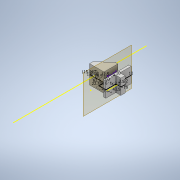
# Autodesk Inventor part: UpperObjectiveMountAssembly
Saved by Autodesk Inventor 2020 (Build 240168000, 168)
## iProperties
Created: 2017-02-08
Part Number: UpperObjectiveMountAssembly
Material: Generic
Document SubType Name: Modeling
Designer: map
Density: 1 g/cm^3
Appearance: Default
Author: map
Autodesk Inventor part; units mm, degrees
ref_plane "XZ Plane" through (0, 0, 0) normal (0, 1, 0) x (-1, 0, 0)
ref_plane "XY Plane" through (0, 0, 0) normal (0, 0, 1) x (1, 0, 0)
sketch "HolePattern" plane through (0, 0, 0) normal (0, 0, 1) x (1, 0, 0)
  arc A0 (32.9386, -36.2368) -> (4.453, -49.3983) centre (80, -175.5) ccw
  arc A1 (1.9216, -50.9498) -> (4.453, -49.3983) centre (4, -51.5) ccw
  arc A2 (1.9216, -50.9498) -> (0, -52.1752) centre (80, -175.5) ccw
  line L0 (0, -52.1752) -> (0, -56)
  line L1 (0, -56) -> (9, -56)
  line L2 (9, -56) -> (24, -56)
  line L3 (24, -56) -> (39, -56)
  line L4 (39, -56) -> (54, -56)
  line L5 (54, -56) -> (69, -56)
  line L6 (69, -56) -> (84, -56)
  line L7 (84, -56) -> (99, -56)
  line L8 (99, -56) -> (108, -56)
  line L9 (108, -56) -> (108, -52.1752)
  arc A3 (108, -52.1752) -> (106.0784, -50.9498) centre (28, -175.5) ccw
  arc A4 (103.547, -49.3983) -> (106.0784, -50.9498) centre (104, -51.5) ccw
  arc A5 (103.547, -49.3983) -> (75.0614, -36.2368) centre (28, -175.5) ccw
  arc A6 (75.0614, -26.7632) -> (75.0614, -36.2368) centre (76.6621, -31.5) ccw
  arc A7 (75.0614, -26.7632) -> (103.547, -13.6017) centre (28, 112.5) ccw
  arc A8 (106.0784, -12.0502) -> (103.547, -13.6017) centre (104, -11.5) ccw
  arc A9 (106.0784, -12.0502) -> (108, -10.8248) centre (28, 112.5) ccw
  line L10 (108, -10.8248) -> (108, 0)
  line L11 (108, 0) -> (0, 0)
  line L12 (0, 0) -> (0, -10.8248)
  arc A10 (0, -10.8248) -> (1.9216, -12.0502) centre (80, 112.5) ccw
  arc A11 (4.453, -13.6017) -> (1.9216, -12.0502) centre (4, -11.5) ccw
  arc A12 (4.453, -13.6017) -> (32.9386, -26.7632) centre (80, 112.5) ccw
  arc A13 (32.9386, -36.2368) -> (32.9386, -26.7632) centre (31.3379, -31.5) ccw
  circle A14 centre (49, -26.5) radius 1.05
  circle A15 centre (59, -36.5) radius 1.05
  circle A16 centre (54, -18.5) radius 1.05
  circle A17 centre (54, -44.5) radius 1.05
  circle A18 centre (59, -21.5) radius 0.75
  circle A19 centre (59, -26.5) radius 0.75
  circle A20 centre (59, -31.5) radius 0.75
  circle A21 centre (59, -41.5) radius 0.75
  circle A22 centre (49, -21.5) radius 0.75
  circle A23 centre (49, -31.5) radius 0.75
  circle A24 centre (49, -36.5) radius 0.75
  circle A25 centre (49, -41.5) radius 0.75
  circle A26 centre (54, -22.5) radius 1.05
  circle A27 centre (54, -40.5) radius 1.05
  circle A28 centre (74, -24) radius 1.25
  circle A29 centre (74, -39) radius 1.25
  circle A30 centre (34, -24) radius 1.25
  circle A31 centre (34, -39) radius 1.25
  circle A32 centre (72.5, -13) radius 1.3
  circle A33 centre (72.5, -50) radius 1.3
  circle A34 centre (35.5, -13) radius 1.3
  circle A35 centre (35.5, -50) radius 1.3
  circle A36 centre (54, -27) radius 1.5
  circle A37 centre (54, -36) radius 1.5
  circle A38 centre (68.5, -24) radius 1.55
  circle A39 centre (68.5, -39) radius 1.55
  circle A40 centre (39.5, -24) radius 1.55
  circle A41 centre (39.5, -39) radius 1.55
  circle A42 centre (61.5, -17) radius 2.8
  circle A43 centre (61.5, -46) radius 2.8
  circle A44 centre (46.5, -17) radius 2.8
  circle A45 centre (46.5, -46) radius 2.8
  circle A46 centre (99, -4) radius 3
  circle A47 centre (84, -4) radius 3
  circle A48 centre (69, -4) radius 3
  circle A49 centre (54, -4) radius 3
  circle A50 centre (39, -4) radius 3
  circle A51 centre (24, -4) radius 3
  circle A52 centre (9, -4) radius 3
  circle A53 centre (39, -46.5) radius 1.3
  circle A54 centre (39, -16.5) radius 1.3
  circle A55 centre (69, -46.5) radius 1.3
  circle A56 centre (69, -16.5) radius 1.3
  circle A57 centre (41.5, -44) radius 1.05
  circle A58 centre (41.5, -31.5) radius 1.05
  circle A59 centre (41.5, -19) radius 1.05
  circle A60 centre (66.5, -44) radius 1.05
  circle A61 centre (66.5, -19) radius 1.05
  circle A62 centre (66.5, -31.5) radius 1.05
  circle A63 centre (44, -41.5) radius 1.05
  circle A64 centre (44, -31.5) radius 1.05
  circle A65 centre (44, -21.5) radius 1.05
  circle A66 centre (64, -41.5) radius 1.05
  circle A67 centre (64, -21.5) radius 1.05
  circle A68 centre (64, -31.5) radius 1.05
  circle A69 centre (46, -34) radius 1
  circle A70 centre (46, -29) radius 1
  circle A71 centre (62, -34) radius 1
  circle A72 centre (62, -29) radius 1
  line L13 (59, -31.5) -> (49, -31.5) construction
  line L14 (54, -36) -> (54, -27) construction
  point P0 (54, -32.5208)
  point P1 (54, -31.5)
sketch "N-565-Profile" plane through (0, 0, 0) normal (0, 0, 1) x (1, 0, 0)
  line L0 (46.2742, 127.3015) -> (66.2742, 127.3015)
  line L1 (66.2742, 127.3015) -> (66.2742, 17.3015)
  line L2 (66.2742, 17.3015) -> (46.2742, 17.3015)
  line L3 (46.2742, 17.3015) -> (46.2742, 127.3015)
  line L4 (46.2742, 127.3015) -> (66.2742, 127.3015) construction
  line L5 (66.2742, 127.3015) -> (66.2742, 140.3015) construction
  line L6 (66.2742, 140.3015) -> (46.2742, 140.3015) construction
  line L7 (46.2742, 140.3015) -> (46.2742, 127.3015) construction
  line L8 (46.2742, 17.3015) -> (66.2742, 17.3015) construction
  line L9 (66.2742, 17.3015) -> (66.2742, 4.3015) construction
  line L10 (66.2742, 4.3015) -> (46.2742, 4.3015) construction
  line L11 (46.2742, 4.3015) -> (46.2742, 17.3015) construction
  point P0 (57.1314, 70.3586)
  point P1 (46.2742, 72.3015)
  dimension "d14" = 20
  dimension "d15" = 110
  dimension "d16" = 13
  dimension "d17" = 13
  measures "d14" distance of L1.end L2.end
  measures "d15" distance of L0.end L1.end
  measures "d16" distance of L5.end L4.end
  measures "d17" distance of L8.end L9.end
sketch "N-565-front-HolePattern" plane through (0, 0, 0) normal (0, 0, 1) x (1, 0, 0)
  circle A0 centre (49, -26.5) radius 1.05
  circle A1 centre (59, -36.5) radius 1.05
  circle A2 centre (54, -18.5) radius 1.05
  circle A3 centre (54, -44.5) radius 1.05
  circle A4 centre (59, -21.5) radius 0.75
  circle A5 centre (59, -26.5) radius 0.75
  circle A6 centre (59, -31.5) radius 0.75
  circle A7 centre (59, -41.5) radius 0.75
  circle A8 centre (49, -21.5) radius 0.75
  circle A9 centre (49, -31.5) radius 0.75
  circle A10 centre (49, -36.5) radius 0.75
  circle A11 centre (49, -41.5) radius 0.75
  circle A12 centre (54, -22.5) radius 1.05
  circle A13 centre (54, -40.5) radius 1.05
  circle A14 centre (74, -24) radius 1.25
  circle A15 centre (74, -39) radius 1.25
  circle A16 centre (34, -24) radius 1.25
  circle A17 centre (34, -39) radius 1.25
  circle A18 centre (72.5, -13) radius 1.3
  circle A19 centre (72.5, -50) radius 1.3
  circle A20 centre (35.5, -13) radius 1.3
  circle A21 centre (35.5, -50) radius 1.3
  circle A22 centre (54, -27) radius 1.5
  circle A23 centre (54, -36) radius 1.5
  circle A24 centre (68.5, -24) radius 1.55
  circle A25 centre (68.5, -39) radius 1.55
  circle A26 centre (39.5, -24) radius 1.55
  circle A27 centre (39.5, -39) radius 1.55
  circle A28 centre (61.5, -17) radius 2.8
  circle A29 centre (61.5, -46) radius 2.8
  circle A30 centre (46.5, -17) radius 2.8
  circle A31 centre (46.5, -46) radius 2.8
  circle A32 centre (39, -46.5) radius 1.3
  circle A33 centre (39, -16.5) radius 1.3
  circle A34 centre (69, -46.5) radius 1.3
  circle A35 centre (69, -16.5) radius 1.3
  circle A36 centre (41.5, -44) radius 1.05
  circle A37 centre (41.5, -31.5) radius 1.05
  circle A38 centre (41.5, -19) radius 1.05
  circle A39 centre (66.5, -44) radius 1.05
  circle A40 centre (66.5, -19) radius 1.05
  circle A41 centre (66.5, -31.5) radius 1.05
  circle A42 centre (44, -41.5) radius 1.05
  circle A43 centre (44, -31.5) radius 1.05
  circle A44 centre (44, -21.5) radius 1.05
  circle A45 centre (64, -41.5) radius 1.05
  circle A46 centre (64, -21.5) radius 1.05
  circle A47 centre (64, -31.5) radius 1.05
  circle A48 centre (46, -34) radius 1
  circle A49 centre (46, -29) radius 1
  circle A50 centre (62, -34) radius 1
  circle A51 centre (62, -29) radius 1
  line L0 (59, -31.5) -> (49, -31.5) construction
  line L1 (54, -36) -> (54, -27) construction
  point P0 (54, -32.5208)
  point P1 (54, -31.5)
derived "__MASTER__.ipt"
sketch "Sketch3" plane through (0, 0, 0) normal (0, 0, 1) x (1, 0, 0)
  line L0 (-12.5, 13) -> (12.5, 13) construction
  line L1 (-12.5, 58) -> (12.5, 58)
  line L2 (0, -289.4339) -> (0, 289.4339)
  line L3 (83, 82.9727) -> (83, 33.0273)
  line L4 (92, 81.3584) -> (92, 34.6416)
  line L5 (12.5, 58) -> (83, 58) construction
  line L6 (-12.5, 79) -> (12.5, 79)
  point P0 (0, 0)
  point P1 (0, 58)
  point P2 (0, 13)
  point P3 (92, 58)
  point P4 (0, 79)
sketch "Profile" plane through (0, 0, 0) normal (0, 0, 1) x (1, 0, 0)
  line L0 (-12.5, 58) -> (12.5, 58) projected
  line L1 (83, 82.9727) -> (83, 33.0273) projected
  line L2 (-12.5, 79) -> (12.5, 79) projected
  line L3 (79.5, 78.9948) -> (99, 78.9948)
  line L4 (99, 78.9948) -> (99, 96.9948)
  line L5 (99, 96.9948) -> (79.5, 96.9948)
  line L6 (77, 145.4948) -> (67, 145.4948)
  line L7 (67, 145.4948) -> (67, 35.4948)
  line L8 (67, 35.4948) -> (77, 35.4948)
  line L9 (77, 35.4948) -> (77, 76.4948)
  line L10 (77, 99.4948) -> (77, 145.4948)
  line L11 (47, 58) -> (-15.5, 58)
  line L12 (-15.5, 58) -> (-15.5, 73.9473)
  line L13 (-15.5, 73.9473) -> (37, 118)
  line L14 (37, 118) -> (47, 118)
  line L15 (47, 118) -> (47, 58)
  line L16 (0, -289.4339) -> (0, 289.4339) projected
  line L17 (37, 118) -> (37, 64) construction
  line L18 (-15.5, 58) -> (47, 58) construction
  line L19 (47, 58) -> (47, 64) construction
  line L20 (47, 64) -> (-15.5, 64) construction
  line L21 (-15.5, 64) -> (-15.5, 58) construction
  arc A0 (77, 99.4948) -> (79.5, 96.9948) centre (79.5, 99.4948) ccw
  arc A1 (79.5, 78.9948) -> (77, 76.4948) centre (79.5, 76.4948) ccw
  circle A2 centre (0, 86.5) radius 6.25
  line L22 (47, 145.4948) -> (67, 145.4948)
  line L23 (67, 145.4948) -> (67, 35.4948)
  line L24 (67, 35.4948) -> (47, 35.4948)
  line L25 (47, 35.4948) -> (47, 145.4948)
  line L26 (47, 145.4948) -> (67, 145.4948) construction
  line L27 (67, 145.4948) -> (67, 158.4948) construction
  line L28 (67, 158.4948) -> (47, 158.4948) construction
  line L29 (47, 158.4948) -> (47, 145.4948) construction
  line L30 (47, 35.4948) -> (67, 35.4948) construction
  line L31 (67, 35.4948) -> (67, 22.4948) construction
  line L32 (67, 22.4948) -> (47, 22.4948) construction
  line L33 (47, 22.4948) -> (47, 35.4948) construction
  dimension "d18" = 18
  dimension "d19" = 10
  dimension "d20" = 6
  dimension "d23" = 130
  dimension "d26" = 10
  dimension "d35" = 62.5
  dimension "d36" = 6
  dimension "d52" = 2.5
  dimension "d53" = 2.5
  dimension "d68" = 43.5
  dimension "d69" = 12.5
  dimension "d70" = 28.5
  dimension "d79" = 22.5052
  dimension "d80" = 60
  dimension "d87" = 22
  dimension "d88" = 15.9473
  constraints: 36 end point, 7 parallel, 6 horizontal, 4 perpendicular, 4 point on circle, 4 tangent, 4 vertical, 3 centre point, 3 point on line, 2 collinear
  measures "d18" distance of L4.end L3.end
  measures "d19" distance of L6.start L6.end
  measures "d20" distance between parallel lines of L1 L9
  measures "d23" angle of L12 L13
  measures "d26" distance of L13.end L14.end
  measures "d35" distance of L11.start L11.end
  measures "d36" distance of L19.end L18.end
  measures "d52" radius of A0
  measures "d53" radius of A1
  measures "d68" distance between parallel lines of L3 L8
  measures "d69" diameter of A2
  measures "d70" distance from line of L11 A2.centre
  measures "d80" distance between parallel lines of L11 L14
  measures "d87" distance between parallel lines of L10 L4
  measures "d88" distance of L11.end L12.end
ref_plane "N-565-front" through (47, 90.4948, 0) normal (1, 0, 0) x (0, 1, 0)
sketch "ObjectiveToN-565-Holes" plane through (47, 90.4948, 0) normal (1, 0, 0) x (0, 1, 0)
  circle A0 centre (-5, 5) radius 1.05
  circle A1 centre (5, -5) radius 1.05
  circle A2 centre (0, 13) radius 1.05
  circle A3 centre (0, -13) radius 1.05
  circle A4 centre (5, 10) radius 0.75
  circle A5 centre (5, 5) radius 0.75
  circle A6 centre (5, 0) radius 0.75
  circle A7 centre (5, -10) radius 0.75
  circle A8 centre (-5, 10) radius 0.75
  circle A9 centre (-5, 0) radius 0.75
  circle A10 centre (-5, -5) radius 0.75
  circle A11 centre (-5, -10) radius 0.75
  circle A12 centre (0, 9) radius 1.05
  circle A13 centre (0, -9) radius 1.05
  circle A14 centre (20, 7.5) radius 1.25
  circle A15 centre (20, -7.5) radius 1.25
  circle A16 centre (-20, 7.5) radius 1.25
  circle A17 centre (-20, -7.5) radius 1.25
  circle A18 centre (18.5, 18.5) radius 1.3
  circle A19 centre (18.5, -18.5) radius 1.3
  circle A20 centre (-18.5, 18.5) radius 1.3
  circle A21 centre (-18.5, -18.5) radius 1.3
  circle A22 centre (0, 4.5) radius 1.5
  circle A23 centre (0, -4.5) radius 1.5
  circle A24 centre (14.5, 7.5) radius 1.55
  circle A25 centre (14.5, -7.5) radius 1.55
  circle A26 centre (-14.5, 7.5) radius 1.55
  circle A27 centre (-14.5, -7.5) radius 1.55
  circle A28 centre (7.5, 14.5) radius 2.8
  circle A29 centre (7.5, -14.5) radius 2.8
  circle A30 centre (-7.5, 14.5) radius 2.8
  circle A31 centre (-7.5, -14.5) radius 2.8
  circle A32 centre (-15, -15) radius 1.3
  circle A33 centre (-15, 15) radius 1.3
  circle A34 centre (15, -15) radius 1.3
  circle A35 centre (15, 15) radius 1.3
  circle A36 centre (-12.5, -12.5) radius 1.05
  circle A37 centre (-12.5, 0) radius 1.05
  circle A38 centre (-12.5, 12.5) radius 1.05
  circle A39 centre (12.5, -12.5) radius 1.05
  circle A40 centre (12.5, 12.5) radius 1.05
  circle A41 centre (12.5, 0) radius 1.05
  circle A42 centre (-10, -10) radius 1.05
  circle A43 centre (-10, 0) radius 1.05
  circle A44 centre (-10, 10) radius 1.05
  circle A45 centre (10, -10) radius 1.05
  circle A46 centre (10, 10) radius 1.05
  circle A47 centre (10, 0) radius 1.05
  circle A48 centre (-8, -2.5) radius 1
  circle A49 centre (-8, 2.5) radius 1
  circle A50 centre (8, -2.5) radius 1
  circle A51 centre (8, 2.5) radius 1
  line L0 (5, 0) -> (-5, 0) construction
  line L1 (0, -4.5) -> (0, 4.5) construction
  point P0 (-90.4948, 0)
  point P1 (0, 0)
  point P2 (0, 0)
  constraints: 1 coincident, 1 other
extrude "ObjectiveMountBody" add sketch "Profile" along normal mid plane 80 contours L11 L12 L13 L2 L16 L0 | L16 A2 L13 L14 L15 L11 L0 | L2 L13 A2 L16 | A2 L13 L16 | L16 L13 A2 picked at (-0.4791, 82.5403) picked at (0.4636, 82.5367)
sketch "Sketch8" plane through (-15.5, 58, 40) normal (-1, 0, 0) x (0, 0, 1)
  line L0 (0, 15.9473) -> (-80, 15.9473) projected
  line L1 (0, 60) -> (0, 15.9473) projected
  line L2 (0, 60) -> (-80, 60) projected
  line L3 (-80, 15.9473) -> (-80, 60) projected
  line L4 (0, 0) -> (-80, 0) projected
  line L5 (0, 15.9473) -> (0, 0) projected
  line L6 (0, 15.9473) -> (-80, 15.9473) projected
  line L7 (-80, 0) -> (-80, 15.9473) projected
  line L8 (0, 60) -> (-80, 60) projected
  line L9 (-74.5, 6) -> (-5.5, 6)
  line L10 (-5.5, 6) -> (-5.5, 60)
  line L11 (-5.5, 60) -> (-74.5, 60)
  line L12 (-74.5, 60) -> (-74.5, 6)
  point P0 (-40, -58)
  dimension "d39" = 6
  dimension "d40" = 5.5
  dimension "d41" = 5.5
  constraints: 8 end point, 2 parallel, 1 horizontal, 1 perpendicular, 1 point on line
  measures "d39" distance between parallel lines of L4 L9
  measures "d40" distance between parallel lines of L3 L12
  measures "d41" distance between parallel lines of L1 L10
extrude "ObjectiveMountHull" cut sketch "Sketch8" against normal blind 52.5 contours L10 L9 L12 L0 | L0 L12 L2 L10
sketch "Sketch9" plane through (-15.5, 64, 34.5) normal (0, 1, 0) x (1, 0, 0)
  point P0 (15.5, 34.5)
hole "Hole1" at (0, 64, 0) direction (0, -1, 0) diameter 20.32 end through all
extrude "MoverToOuterBracket" add sketch "Profile" along normal mid plane 65 separate body contours L7 L6 L10 A0 L5 L4 L3 A1 L9 L8
sketch "BracketHoles" plane through (67, 35.4948, 32.5) normal (-1, 0, 0) x (0, 0, 1)
  line L0 (-65, 0) -> (-65, 110) projected
  line L1 (-65, 110) -> (0, 110) projected
  line L2 (0, 110) -> (0, 0) projected
  line L3 (0, 0) -> (-65, 0) projected
  line L4 (-65, 55) -> (0, 55)
  line L5 (-32.5, 110) -> (-32.5, 0)
  line L6 (0, 0) -> (-65, 0) projected
  line L7 (-47, 62.5) -> (-18, 62.5) construction
  line L8 (-18, 62.5) -> (-18, 47.5) construction
  line L9 (-18, 47.5) -> (-47, 47.5) construction
  line L10 (-47, 47.5) -> (-47, 62.5) construction
  line L11 (-45, 105) -> (-20, 105) construction
  line L12 (-20, 105) -> (-20, 5) construction
  line L13 (-20, 5) -> (-45, 5) construction
  line L14 (-45, 5) -> (-45, 105) construction
  line L15 (-32.5, 59.5) -> (-32.5, 50.5) construction
  point P0 (-32.5, -35.4948)
  point P1 (-47, 55)
  point P2 (-32.5, 62.5)
  point P3 (-45, 55)
  point P4 (-32.5, 105)
  point P5 (-32.5, 105)
  point P6 (-32.5, 5)
  point P7 (-32.5, 55)
  dimension "d56" = 29
  dimension "d57" = 15
  dimension "d58" = 25
  dimension "d59" = 100
  dimension "d60" = 9
  constraints: 22 end point, 11 coincident, 11 midpoint, 4 parallel, 4 point on line, 2 horizontal, 2 perpendicular, 1 collinear, 1 vertical
  measures "d56" distance of L8.end L9.end
  measures "d57" distance of L7.end L8.end
  measures "d58" distance of L12.end L13.end
  measures "d59" distance of L11.end L12.end
  measures "d60" distance of L15.start L15.end
sketch "Sketch12" plane through (37, 58, 40) normal (-1, 0, 0) x (0, 0, 1)
  arc A0 (-50, 50) -> (-30, 50) centre (-40, 50) ccw
  line L0 (-5.5, 60) -> (-74.5, 60) projected
  line L1 (-50, 50) -> (-50, 60)
  line L2 (0, 60) -> (-80, 60) projected
  line L3 (-30, 50) -> (-30, 60)
  line L4 (-40, 60) -> (-40, 50) construction
  point P0 (-40, -58)
  dimension "d61" = 20
  dimension "d62" = 10
  constraints: 6 end point, 2 perpendicular, 2 point on circle, 2 point on line, 2 tangent, 1 centre point, 1 midpoint, 1 vertical
  measures "d61" diameter of A0
  measures "d62" distance from line of L0 L4.end
extrude "LensMountClearance" cut sketch "Sketch12" against normal through all bodies 1
chamfer "Chamfer1" distance 7 angle 45 2 edges at (42, 118, -10) (42, 118, 10)
extrude "Extrusion8" cut sketch "Profile" against normal through all contours A2 L13 L16 | L16 L13 A2 | A2 L16 L13 | L16 A2 L13 bodies 1
chamfer "Chamfer3" distance 2 angle 45 2 edges at (4.5572, 90.7772, -37.25) (-5.0036, 82.7548, -37.25)
